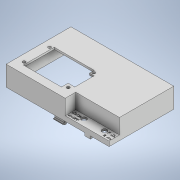
# Autodesk Inventor part: housing top
Saved by Autodesk Inventor 2020 (Build 240168000, 168)
## iProperties
Created: 2019-10-19
Part Number: housing top
Material: Generic
Document SubType Name: Modeling
Designer: strom
Density: 1 g/cm^3
Appearance: Default
Author: strom
Autodesk Inventor part; units mm, degrees
note: some values were not read from the file. Chosen so that the rebuilt part matches the saved one: direction of "Emboss1".
ref_plane "YZ Plane" through (0, 0, 0) normal (1, 0, 0) x (0, 1, 0)
ref_plane "XZ Plane" through (0, 0, 0) normal (0, 1, 0) x (-1, 0, 0)
sketch "Sketch1" plane through (0, 0, 0) normal (0, 1, 0) x (-1, 0, 0)
  line L0 (68.58, 43.18) -> (-68.58, 43.18)
  line L1 (-68.58, 43.18) -> (-68.58, -43.18)
  line L2 (-68.58, -43.18) -> (68.58, -43.18)
  line L3 (68.58, -43.18) -> (68.58, 43.18)
  line L4 (68.58, 43.18) -> (-68.58, -43.18) construction
  line L5 (-68.58, 43.18) -> (68.58, -43.18) construction
  point P0 (0, 0)
  dimension "d0" = 137.16
  dimension "d1" = 86.36
  constraints: 12 end point, 2 midpoint, 2 parallel, 1 horizontal, 1 perpendicular
  measures "d0" distance of L2.end L1.end
  measures "d1" distance of L1.end L0.end
extrude "Extrusion1" add sketch "Sketch1" along normal blind 25.4
sketch "Sketch2" plane through (0, 25.4, 0) normal (0, 1, 0) x (1, 0, 0)
  line L0 (-68.58, -43.18) -> (68.58, -43.18) projected
  line L1 (68.58, -43.18) -> (10.16, -43.18)
  line L2 (10.16, -43.18) -> (10.16, -29.21)
  line L3 (10.16, -29.21) -> (68.58, -29.21)
  line L4 (68.58, -29.21) -> (68.58, -43.18)
  point P0 (0, 0)
  dimension "d4" = 58.42
  dimension "d5" = 13.97
  constraints: 8 end point, 2 parallel, 1 horizontal, 1 perpendicular
  measures "d4" distance of L2.end L3.end
  measures "d5" distance of L1.end L2.end
extrude "Extrusion2" cut sketch "Sketch2" against normal blind 20.193
shell "Shell1" thickness 2.54 removed faces 1 at (-22.86, 0, -14.3933)
sketch "Sketch3" plane through (0, 0, 0) normal (0, -1, 0) x (1, 0, 0)
  line L0 (66.04, 40.64) -> (66.04, -40.64) projected
  line L1 (66.04, -40.64) -> (-66.04, -40.64) projected
  line L2 (-66.04, -40.64) -> (-66.04, 40.64) projected
  line L3 (-66.04, 40.64) -> (66.04, 40.64) projected
  line L4 (68.58, -43.18) -> (-68.58, -43.18) projected
  line L5 (68.58, 43.18) -> (68.58, -43.18) projected
  line L6 (-68.58, 43.18) -> (68.58, 43.18) projected
  line L7 (-68.58, -43.18) -> (-68.58, 43.18) projected
  line L8 (67.31, -41.91) -> (-67.31, -41.91)
  line L9 (-67.31, -41.91) -> (-67.31, 41.91)
  line L10 (-67.31, 41.91) -> (67.31, 41.91)
  line L11 (67.31, 41.91) -> (67.31, -41.91)
  line L12 (67.31, -41.91) -> (-67.31, 41.91) construction
  line L13 (-67.31, -41.91) -> (67.31, 41.91) construction
  point P0 (0, 0)
  dimension "d9" = 1.27
  dimension "d10" = 1.27
  constraints: 12 end point, 2 midpoint, 2 parallel, 1 horizontal, 1 perpendicular
  measures "d9" distance between parallel lines of L9 L2
  measures "d10" distance between parallel lines of L6 L10
extrude "Extrusion3" add sketch "Sketch3" along normal blind 1.27 contours L4 L7 L6 L5
sketch "Sketch4" plane through (0, -1.27, 0) normal (0, -1, 0) x (1, 0, 0)
  line L0 (68.58, 43.18) -> (-68.58, 43.18) projected
  line L1 (-66.04, 40.64) -> (66.04, 40.64) projected
  line L2 (36.449, 43.18) -> (43.688, 43.18)
  line L3 (43.688, 43.18) -> (43.688, 40.64)
  line L4 (43.688, 40.64) -> (36.449, 40.64)
  line L5 (36.449, 40.64) -> (36.449, 43.18)
  line L6 (68.58, -43.18) -> (68.58, 43.18) projected
  point P0 (0, 0)
  dimension "d13" = 24.892
  dimension "d14" = 7.239
  constraints: 8 end point, 2 parallel, 2 point on line, 1 horizontal, 1 perpendicular
  measures "d13" distance from line of L6 L3.end
  measures "d14" distance between parallel lines of L3 L5
extrude "Extrusion4" add sketch "Sketch4" along normal blind 3.81 and the other way blind 1.27
sketch "Sketch5" plane through (0, 0, 0) normal (1, 0, 0) x (0, 1, 0)
  line L0 (0, 40.64) -> (22.86, 40.64) projected
  line L1 (22.86, 40.64) -> (22.86, 37.846)
  line L2 (22.86, 40.64) -> (25.654, 40.64) construction
  line L3 (22.86, 37.846) -> (-8.89, 37.846)
  line L4 (-8.89, 37.846) -> (-8.89, 40.132)
  line L5 (-8.89, 40.132) -> (-7.2004, 42.545)
  line L6 (-7.2004, 42.545) -> (-6.35, 42.545)
  line L7 (-6.35, 42.545) -> (-6.35, 40.386)
  line L8 (-6.35, 40.386) -> (0, 40.386)
  line L9 (0, -40.64) -> (0, 40.64) projected
  line L10 (-1.27, 43.18) -> (25.4, 43.18) projected
  line L11 (-1.27, 43.18) -> (-1.27, -43.18) projected
  line L12 (0, 41.91) -> (0, -41.91) projected
  line L13 (22.86, -40.64) -> (22.86, 40.64) projected
  point P0 (0, 0)
  dimension "d21" = 2.54
  dimension "d22" = 0.254
  dimension "d23" = 35
  dimension "d25" = 5.08
  dimension "d26" = 2.54
  dimension "d31" = 0.508
  dimension "d32" = 1.905
  constraints: 16 end point, 3 perpendicular, 2 parallel, 2 point on line, 1 collinear, 1 horizontal, 1 vertical
  measures "d21" distance between parallel lines of L3 L8
  measures "d22" distance between parallel lines of L0 L8
  measures "d23" angle of L4 L5
  measures "d25" distance between parallel lines of L11 L7
  measures "d26" distance between parallel lines of L7 L4
  measures "d31" distance from line of L0 L4.end
  measures "d32" distance between parallel lines of L6 L0
extrude "Extrusion5" add sketch "Sketch5" along normal mid plane 12.7
ref_plane "Work Plane1" through (33.274, 5.207, 29.21) normal (1, 0, 0) x (0, 0, -1)
sketch "Sketch6" plane through (33.274, 5.207, 29.21) normal (1, 0, 0) x (0, 0, -1)
  line L0 (-13.97, -6.477) -> (-13.97, 20.193) projected
  line L1 (72.39, 20.193) -> (-13.97, 20.193) projected
  line L2 (72.39, -6.477) -> (72.39, 20.193) projected
  line L3 (-13.97, -6.477) -> (72.39, -6.477) projected
  line L4 (-12.7, -5.207) -> (71.12, -5.207) projected
  line L5 (71.12, -5.207) -> (71.12, -6.477) projected
  line L6 (69.85, -5.207) -> (69.85, 17.653) projected
  line L7 (67.056, 17.653) -> (67.056, -14.097)
  line L8 (67.056, -14.097) -> (69.342, -14.097)
  line L9 (69.342, -14.097) -> (71.755, -12.4074)
  line L10 (71.755, -12.4074) -> (71.755, -11.5692)
  line L11 (71.755, -11.5692) -> (69.596, -11.5692)
  line L12 (69.596, -11.5692) -> (69.596, -5.207)
  line L13 (69.85, 17.653) -> (-11.43, 17.653) projected
  point P0 (29.21, -5.207)
  dimension "d34" = 0.254
  dimension "d35" = 35
  dimension "d36" = 2.794
  dimension "d38" = 2.286
  dimension "d39" = 4.699
  dimension "d40" = 0.8382
  dimension "d41" = 31.75
  constraints: 12 end point, 3 perpendicular, 2 point on line, 1 parallel, 1 vertical
  measures "d34" distance between parallel lines of L6 L12
  measures "d35" angle of L8 L9
  measures "d36" distance between parallel lines of L7 L6
  measures "d38" distance of L7.end L8.end
  measures "d39" distance between parallel lines of L10 L7
  measures "d40" distance of L9.end L10.end
  measures "d41" distance of L7.start L7.end
extrude "Extrusion6" add sketch "Sketch6" along normal mid plane 12.7 contours L7 L4 L12 L3 | L3 L12 L11 L10 L9 L8 L7 | L7 L13 L6 L4
sketch "Sketch7" plane through (0, 5.207, 0) normal (0, 1, 0) x (1, 0, 0)
  line L0 (68.58, -29.21) -> (68.58, -43.18) projected
  line L1 (10.16, -29.21) -> (68.58, -29.21) projected
  line L2 (10.16, -43.18) -> (10.16, -29.21) projected
  line L3 (68.58, -43.18) -> (10.16, -43.18) projected
  circle A0 centre (26.416, -34.3535) radius 3.2385
  circle A1 centre (53.721, -34.3535) radius 3.2385
  line L4 (68.58, -43.18) -> (10.16, -43.18) projected
  line L5 (36.449, -43.18) -> (36.449, -40.64) projected
  line L6 (36.449, -40.64) -> (43.688, -40.64) projected
  line L7 (43.688, -40.64) -> (43.688, -43.18) projected
  line L8 (43.688, -43.18) -> (36.449, -43.18) projected
  point P0 (0, 0)
  dimension "d44" = 6.477
  dimension "d45" = 6.477
  dimension "d46" = 27.305
  dimension "d47" = 10.033
  dimension "d48" = 8.8265
  constraints: 2 centre point, 1 horizontal alignment
  measures "d44" diameter of A0
  measures "d45" diameter of A1
  measures "d46" distance of A1.centre A0.centre
  measures "d47" distance from line of A1.centre L7
  measures "d48" distance from line of L3 A1.centre
extrude "Extrusion7" cut sketch "Sketch7" against normal blind 12.7 contours A0 | A1
sketch "Sketch8" plane through (0, 25.4, 0) normal (0, 1, 0) x (1, 0, 0)
  line L0 (10.16, -43.18) -> (10.16, -29.21) projected
  line L1 (10.16, -29.21) -> (68.58, -29.21) projected
  line L2 (68.58, -29.21) -> (68.58, 43.18) projected
  line L3 (68.58, 43.18) -> (-68.58, 43.18) projected
  line L4 (-68.58, 43.18) -> (-68.58, -43.18) projected
  line L5 (-68.58, -43.18) -> (10.16, -43.18) projected
  line L6 (-66.04, -40.64) -> (-6.35, -40.64) projected
  line L7 (39.624, 37.846) -> (39.624, 40.64) projected
  line L8 (66.04, 40.64) -> (39.624, 40.64) projected
  line L9 (66.04, -26.67) -> (66.04, 40.64) projected
  line L10 (7.62, -26.67) -> (66.04, -26.67) projected
  line L11 (7.62, -40.64) -> (7.62, -26.67) projected
  line L12 (6.35, -40.64) -> (7.62, -40.64) projected
  line L13 (6.35, -40.64) -> (6.35, -37.846) projected
  line L14 (6.35, -37.846) -> (-6.35, -37.846) projected
  line L15 (-6.35, -37.846) -> (-6.35, -40.64) projected
  line L16 (-66.04, -40.64) -> (-6.35, -40.64) projected
  line L17 (-66.04, 40.64) -> (-66.04, -40.64) projected
  line L18 (26.924, 40.64) -> (-66.04, 40.64) projected
  line L19 (26.924, 40.64) -> (26.924, 37.846) projected
  line L20 (26.924, 37.846) -> (39.624, 37.846) projected
  line L21 (-64.77, 9.652) -> (4.826, 9.652)
  line L22 (4.826, 9.652) -> (4.826, -34.036)
  line L23 (4.826, -34.036) -> (-64.77, -34.036)
  line L24 (-64.77, -34.036) -> (-64.77, 9.652)
  line L25 (-56.134, 9.652) -> (-56.134, -34.036)
  line L26 (-2.794, 9.652) -> (-2.794, 2.032)
  line L27 (-2.794, 2.032) -> (4.826, 2.032)
  line L28 (-5.334, -34.036) -> (-5.334, -23.876)
  line L29 (-5.334, -23.876) -> (4.826, -23.876)
  line L30 (-5.334, -32.766) -> (-56.134, -32.766)
  line L31 (-56.134, 8.382) -> (-2.794, 8.382)
  line L32 (3.556, 2.032) -> (3.556, -23.876)
  point P0 (0, 0)
  dimension "d51" = 3.81
  dimension "d52" = 3.81
  dimension "d53" = 43.688
  dimension "d54" = 69.596
  dimension "d55" = 8.636
  dimension "d56" = 1.27
  dimension "d57" = 1.27
  dimension "d58" = 10.16
  dimension "d59" = 10.16
  dimension "d60" = 1.27
  dimension "d61" = 7.62
  dimension "d62" = 7.62
  constraints: 24 end point, 12 point on line, 7 perpendicular, 2 parallel, 2 vertical, 1 horizontal
  measures "d51" distance between parallel lines of L4 L24
  measures "d52" distance between parallel lines of L23 L14
  measures "d53" distance between parallel lines of L21 L23
  measures "d54" distance between parallel lines of L22 L24
  measures "d55" distance between parallel lines of L24 L25
  measures "d56" distance between parallel lines of L21 L31
  measures "d57" distance between parallel lines of L23 L30
  measures "d58" distance between parallel lines of L23 L29
  measures "d59" distance between parallel lines of L28 L22
  measures "d60" distance between parallel lines of L32 L22
  measures "d61" distance between parallel lines of L27 L21
  measures "d62" distance between parallel lines of L22 L26
extrude "Extrusion8" cut sketch "Sketch8" against normal blind 12.7 contours L31 L26 L27 L32 L29 L28 L30 L25
sketch "Sketch9" plane through (0, 25.4, 0) normal (0, 1, 0) x (1, 0, 0)
  circle A0 centre (-0.254, 5.207) radius 1.905
  circle A1 centre (-0.254, -28.829) radius 1.905
  circle A2 centre (-59.182, -28.829) radius 1.905
  circle A3 centre (-59.182, 5.207) radius 1.905
  line L0 (-2.794, 2.032) -> (3.556, 2.032) projected
  line L1 (-2.794, 8.382) -> (-2.794, 2.032) projected
  point P0 (0, 0)
  dimension "d65" = 3.81
  dimension "d66" = 3.81
  dimension "d67" = 3.81
  dimension "d68" = 3.81
  dimension "d69" = 58.928
  dimension "d70" = 34.036
  dimension "d71" = 3.175
  dimension "d72" = 2.54
  constraints: 4 centre point, 2 horizontal alignment, 2 vertical alignment
  measures "d65" diameter of A3
  measures "d66" diameter of A2
  measures "d67" diameter of A0
  measures "d68" diameter of A1
  measures "d69" distance of A0.centre A3.centre
  measures "d70" distance of A2.centre A3.centre
  measures "d71" distance from line of A0.centre L0
  measures "d72" distance from line of A0.centre L1
extrude "Extrusion9" cut sketch "Sketch9" against normal blind 12.7
sketch "Sketch10" plane through (0, 5.207, 0) normal (0, 1, 0) x (1, 0, 0)
  line L0 (11.43, -34.29) -> (13.0175, -34.29)
  line L1 (13.0175, -34.29) -> (13.0175, -32.385)
  line L2 (13.0175, -32.385) -> (14.9225, -32.385)
  line L3 (14.9225, -32.385) -> (14.9225, -34.29)
  line L4 (14.9225, -34.29) -> (16.51, -34.29)
  line L5 (16.51, -34.29) -> (16.51, -35.56)
  line L6 (16.51, -35.56) -> (11.43, -35.56)
  line L7 (11.43, -35.56) -> (11.43, -34.29)
  line L8 (11.43, -40.8622) -> (16.51, -40.8622)
  line L9 (16.51, -40.8622) -> (16.51, -39.5922)
  line L10 (16.51, -39.5922) -> (14.9225, -39.5922)
  line L11 (14.9225, -39.5922) -> (14.9225, -39.116)
  line L12 (14.9225, -39.116) -> (13.0175, -39.116)
  line L13 (13.0175, -39.116) -> (13.0175, -39.5922)
  line L14 (13.0175, -39.5922) -> (11.43, -39.5922)
  line L15 (11.43, -40.8622) -> (11.43, -39.5922)
  line L16 (10.16, -43.18) -> (10.16, -29.21) projected
  line L17 (10.16, -29.21) -> (68.58, -29.21) projected
  line L18 (14.661, -39.3775) -> (14.661, -39.8537)
  line L19 (14.661, -39.8537) -> (16.2485, -39.8537)
  line L20 (16.2485, -39.8537) -> (16.2485, -40.6008)
  line L21 (16.2485, -40.6008) -> (11.6915, -40.6008)
  line L22 (11.6915, -40.6008) -> (11.6915, -39.8537)
  line L23 (11.6915, -39.8537) -> (13.279, -39.8537)
  line L24 (13.279, -39.8537) -> (13.279, -39.3775)
  line L25 (13.279, -39.3775) -> (14.661, -39.3775)
  line L26 (16.2537, -34.5463) -> (14.6662, -34.5463)
  line L27 (14.6662, -34.5463) -> (14.6662, -32.6413)
  line L28 (14.6662, -32.6413) -> (13.2738, -32.6413)
  line L29 (13.2738, -32.6413) -> (13.2738, -34.5463)
  line L30 (13.2738, -34.5463) -> (11.6863, -34.5463)
  line L31 (11.6863, -34.5463) -> (11.6863, -35.3037)
  line L32 (11.6863, -35.3037) -> (16.2537, -35.3037)
  line L33 (16.2537, -35.3037) -> (16.2537, -34.5463)
  line L34 (17.0101, -32.6962) -> (22.7751, -32.6962) construction
  line L35 (22.7751, -32.6962) -> (22.7751, -35.8726) construction
  line L36 (22.7751, -35.8726) -> (17.0101, -35.8726) construction
  line L37 (17.0101, -35.8726) -> (17.0101, -32.6962) construction
  line L38 (17.0101, -38.1814) -> (22.4449, -38.1814) construction
  line L39 (22.4449, -38.1814) -> (22.4449, -41.4779) construction
  line L40 (22.4449, -41.4779) -> (17.0101, -41.4779) construction
  line L41 (17.0101, -41.4779) -> (17.0101, -38.1814) construction
  line L42 (62.753, -34.29) -> (64.3405, -34.29)
  line L43 (64.3405, -34.29) -> (64.3405, -32.385)
  line L44 (64.3405, -32.385) -> (66.2455, -32.385)
  line L45 (66.2455, -32.385) -> (66.2455, -34.29)
  line L46 (66.2455, -34.29) -> (67.833, -34.29)
  line L47 (67.833, -34.29) -> (67.833, -35.56)
  line L48 (67.833, -35.56) -> (62.753, -35.56)
  line L49 (62.753, -35.56) -> (62.753, -34.29)
  line L50 (12.925, -32.9588) -> (11.3375, -32.9588)
  line L51 (66.2455, -39.116) -> (66.2455, -39.5922)
  line L52 (64.3405, -39.116) -> (66.2455, -39.116)
  line L53 (62.753, -40.8622) -> (62.753, -39.5922)
  line L54 (62.753, -39.5922) -> (64.3405, -39.5922)
  line L55 (67.833, -40.8622) -> (62.753, -40.8622)
  line L56 (66.2455, -39.5922) -> (67.833, -39.5922)
  line L57 (64.3405, -39.5922) -> (64.3405, -39.116)
  line L58 (67.833, -39.5922) -> (67.833, -40.8622)
  line L59 (67.579, -34.544) -> (65.9915, -34.544)
  line L60 (65.9915, -34.544) -> (65.9915, -32.639)
  line L61 (65.9915, -32.639) -> (64.5945, -32.639)
  line L62 (64.5945, -32.639) -> (64.5945, -34.544)
  line L63 (64.5945, -34.544) -> (63.007, -34.544)
  line L64 (63.007, -34.544) -> (63.007, -35.306)
  line L65 (63.007, -35.306) -> (67.579, -35.306)
  line L66 (67.579, -35.306) -> (67.579, -34.544)
  line L67 (67.579, -39.8462) -> (65.9915, -39.8462)
  line L68 (65.9915, -39.8462) -> (65.9915, -39.37)
  line L69 (65.9915, -39.37) -> (64.5945, -39.37)
  line L70 (64.5945, -39.37) -> (64.5945, -39.8462)
  line L71 (64.5945, -39.8462) -> (63.007, -39.8462)
  line L72 (63.007, -39.8462) -> (63.007, -40.6082)
  line L73 (63.007, -40.6082) -> (67.579, -40.6082)
  line L74 (67.579, -40.6082) -> (67.579, -39.8462)
  line L75 (58.0602, -32.1559) -> (60.2461, -32.1559) construction
  line L76 (60.2461, -32.1559) -> (60.2461, -35.2039) construction
  line L77 (60.2461, -35.2039) -> (58.0602, -35.2039) construction
  line L78 (58.0602, -35.2039) -> (58.0602, -32.1559) construction
  line L79 (58.0602, -38.2294) -> (60.6611, -38.2294) construction
  line L80 (60.6611, -38.2294) -> (60.6611, -41.2774) construction
  line L81 (60.6611, -41.2774) -> (58.0602, -41.2774) construction
  line L82 (58.0602, -41.2774) -> (58.0602, -38.2294) construction
  spline S0 degree 2 poles (19.4752, -33.1087) (19.6481, -33.3112) (19.8407, -33.904) (19.8407, -34.2844) knots 0 0 0 1 2 2 2
  spline S1 degree 2 poles (19.8407, -34.2844) (19.8407, -34.6549) (19.653, -35.2551) (19.4752, -35.4576) knots 0 0 0 1 2 2 2
  spline S2 degree 2 poles (19.4752, -35.4576) (19.2875, -35.6701) (18.791, -35.8726) (18.4921, -35.8726) knots 0 0 0 1 2 2 2
  spline S3 degree 2 poles (18.4921, -35.8726) (18.1834, -35.8726) (17.6894, -35.6627) (17.5091, -35.4576) knots 0 0 0 1 2 2 2
  spline S4 degree 2 poles (17.5091, -35.4576) (17.3337, -35.2551) (17.146, -34.6598) (17.146, -34.2844) knots 0 0 0 1 2 2 2
  spline S5 degree 2 poles (17.146, -34.2844) (17.146, -33.9015) (17.3361, -33.3186) (17.5115, -33.1087) knots 0 0 0 1 2 2 2
  spline S6 degree 2 poles (17.5115, -33.1087) (17.6894, -32.9061) (18.1858, -32.6962) (18.4921, -32.6962) knots 0 0 0 1 2 2 2
  spline S7 degree 2 poles (18.4921, -32.6962) (18.8033, -32.6962) (19.3023, -32.9135) (19.4752, -33.1087) knots 0 0 0 1 2 2 2
  spline S8 degree 2 poles (19.4184, -34.2844) (19.4184, -33.983) (19.2875, -33.5162) (19.1689, -33.3631) knots 0 0 0 1 2 2 2
  spline S9 degree 2 poles (19.1689, -33.3631) (19.0479, -33.205) (18.707, -33.0469) (18.4946, -33.0469) knots 0 0 0 1 2 2 2
  spline S10 degree 2 poles (18.4946, -33.0469) (18.2748, -33.0469) (17.9438, -33.2001) (17.8178, -33.3631) knots 0 0 0 1 2 2 2
  spline S11 degree 2 poles (17.8178, -33.3631) (17.6968, -33.5187) (17.5683, -33.988) (17.5683, -34.2844) knots 0 0 0 1 2 2 2
  spline S12 degree 2 poles (17.5683, -34.2844) (17.5683, -34.8846) (18.0722, -35.5219) (18.4946, -35.5219) knots 0 0 0 1 2 2 2
  spline S13 degree 2 poles (18.4946, -35.5219) (18.917, -35.5219) (19.4184, -34.8846) (19.4184, -34.2844) knots 0 0 0 1 2 2 2
  line L83 (22.4664, -35.8084) -> (22.0119, -35.8084)
  line L84 (22.0119, -35.8084) -> (20.6633, -33.1803)
  line L85 (20.6633, -33.1803) -> (20.6633, -35.8084)
  line L86 (20.6633, -35.8084) -> (20.2853, -35.8084)
  line L87 (20.2853, -35.8084) -> (20.2853, -32.7604)
  line L88 (20.2853, -32.7604) -> (20.8609, -32.7604)
  line L89 (20.8609, -32.7604) -> (22.0885, -35.1736)
  line L90 (22.0885, -35.1736) -> (22.0885, -32.7604)
  line L91 (22.0885, -32.7604) -> (22.4664, -32.7604)
  line L92 (22.4664, -32.7604) -> (22.4664, -35.8084)
  spline S14 degree 2 poles (19.4752, -38.5939) (19.6481, -38.7964) (19.8407, -39.3892) (19.8407, -39.7696) knots 0 0 0 1 2 2 2
  spline S15 degree 2 poles (19.8407, -39.7696) (19.8407, -40.1401) (19.653, -40.7403) (19.4752, -40.9429) knots 0 0 0 1 2 2 2
  spline S16 degree 2 poles (19.4752, -40.9429) (19.2875, -41.1553) (18.791, -41.3578) (18.4921, -41.3578) knots 0 0 0 1 2 2 2
  spline S17 degree 2 poles (18.4921, -41.3578) (18.1834, -41.3578) (17.6894, -41.1479) (17.5091, -40.9429) knots 0 0 0 1 2 2 2
  spline S18 degree 2 poles (17.5091, -40.9429) (17.3337, -40.7403) (17.146, -40.1451) (17.146, -39.7696) knots 0 0 0 1 2 2 2
  spline S19 degree 2 poles (17.146, -39.7696) (17.146, -39.3868) (17.3361, -38.8038) (17.5115, -38.5939) knots 0 0 0 1 2 2 2
  spline S20 degree 2 poles (17.5115, -38.5939) (17.6894, -38.3913) (18.1858, -38.1814) (18.4921, -38.1814) knots 0 0 0 1 2 2 2
  spline S21 degree 2 poles (18.4921, -38.1814) (18.8033, -38.1814) (19.3023, -38.3988) (19.4752, -38.5939) knots 0 0 0 1 2 2 2
  spline S22 degree 2 poles (19.4184, -39.7696) (19.4184, -39.4683) (19.2875, -39.0014) (19.1689, -38.8483) knots 0 0 0 1 2 2 2
  spline S23 degree 2 poles (19.1689, -38.8483) (19.0479, -38.6902) (18.707, -38.5321) (18.4946, -38.5321) knots 0 0 0 1 2 2 2
  spline S24 degree 2 poles (18.4946, -38.5321) (18.2748, -38.5321) (17.9438, -38.6853) (17.8178, -38.8483) knots 0 0 0 1 2 2 2
  spline S25 degree 2 poles (17.8178, -38.8483) (17.6968, -39.0039) (17.5683, -39.4732) (17.5683, -39.7696) knots 0 0 0 1 2 2 2
  spline S26 degree 2 poles (17.5683, -39.7696) (17.5683, -40.3698) (18.0722, -41.0071) (18.4946, -41.0071) knots 0 0 0 1 2 2 2
  spline S27 degree 2 poles (18.4946, -41.0071) (18.917, -41.0071) (19.4184, -40.3698) (19.4184, -39.7696) knots 0 0 0 1 2 2 2
  line L93 (22.1082, -38.6062) -> (20.6904, -38.6062)
  line L94 (20.6904, -38.6062) -> (20.6904, -39.4658)
  line L95 (20.6904, -39.4658) -> (22.0489, -39.4658)
  line L96 (22.0489, -39.4658) -> (22.0489, -39.8264)
  line L97 (22.0489, -39.8264) -> (20.6904, -39.8264)
  line L98 (20.6904, -39.8264) -> (20.6904, -41.2936)
  line L99 (20.6904, -41.2936) -> (20.2853, -41.2936)
  line L100 (20.2853, -41.2936) -> (20.2853, -38.2456)
  line L101 (20.2853, -38.2456) -> (22.1082, -38.2456)
  line L102 (22.1082, -38.2456) -> (22.1082, -38.6062)
  line L103 (24.2942, -38.6062) -> (22.8764, -38.6062)
  line L104 (22.8764, -38.6062) -> (22.8764, -39.4658)
  line L105 (22.8764, -39.4658) -> (24.2349, -39.4658)
  line L106 (24.2349, -39.4658) -> (24.2349, -39.8264)
  line L107 (24.2349, -39.8264) -> (22.8764, -39.8264)
  line L108 (22.8764, -39.8264) -> (22.8764, -41.2936)
  line L109 (22.8764, -41.2936) -> (22.4713, -41.2936)
  line L110 (22.4713, -41.2936) -> (22.4713, -38.2456)
  line L111 (22.4713, -38.2456) -> (24.2942, -38.2456)
  line L112 (24.2942, -38.2456) -> (24.2942, -38.6062)
  line L113 (60.1918, -32.5165) -> (58.774, -32.5165)
  line L114 (58.774, -32.5165) -> (58.774, -33.376)
  line L115 (58.774, -33.376) -> (60.1325, -33.376)
  line L116 (60.1325, -33.376) -> (60.1325, -33.7367)
  line L117 (60.1325, -33.7367) -> (58.774, -33.7367)
  line L118 (58.774, -33.7367) -> (58.774, -35.2039)
  line L119 (58.774, -35.2039) -> (58.3689, -35.2039)
  line L120 (58.3689, -35.2039) -> (58.3689, -32.1559)
  line L121 (58.3689, -32.1559) -> (60.1918, -32.1559)
  line L122 (60.1918, -32.1559) -> (60.1918, -32.5165)
  line L123 (60.7278, -41.2774) -> (60.2017, -41.2774)
  line L124 (60.2017, -41.2774) -> (59.2384, -40.0647)
  line L125 (59.2384, -40.0647) -> (58.774, -40.0647)
  line L126 (58.774, -40.0647) -> (58.774, -41.2774)
  line L127 (58.774, -41.2774) -> (58.3689, -41.2774)
  line L128 (58.3689, -41.2774) -> (58.3689, -38.2294)
  line L129 (58.3689, -38.2294) -> (59.1544, -38.2294)
  spline S28 degree 2 poles (59.1544, -38.2294) (59.4162, -38.2294) (59.7694, -38.2863) (59.93, -38.39) knots 0 0 0 1 2 2 2
  spline S29 degree 2 poles (59.93, -38.39) (60.0905, -38.4937) (60.2758, -38.8173) (60.2758, -39.0569) knots 0 0 0 1 2 2 2
  spline S30 degree 2 poles (60.2758, -39.0569) (60.2758, -39.3904) (59.9349, -39.8424) (59.6434, -39.951) knots 0 0 0 1 2 2 2
  line L130 (59.6434, -39.951) -> (60.7278, -41.2774)
  spline S31 degree 2 poles (59.8534, -39.089) (59.8534, -38.9556) (59.7595, -38.7506) (59.6607, -38.6839) knots 0 0 0 1 2 2 2
  spline S32 degree 2 poles (59.6607, -38.6839) (59.5743, -38.6271) (59.3446, -38.5802) (59.1766, -38.5802) knots 0 0 0 1 2 2 2
  line L131 (59.1766, -38.5802) -> (58.774, -38.5802)
  line L132 (58.774, -38.5802) -> (58.774, -39.7263)
  line L133 (58.774, -39.7263) -> (59.1297, -39.7263)
  spline S33 degree 2 poles (59.1297, -39.7263) (59.305, -39.7263) (59.5842, -39.6645) (59.6805, -39.5682) knots 0 0 0 1 2 2 2
  spline S34 degree 2 poles (59.6805, -39.5682) (59.7694, -39.4842) (59.8534, -39.2471) (59.8534, -39.089) knots 0 0 0 1 2 2 2
  point P0 (0, 0)
  point P1 (13.0175, -39.3541)
  point P2 (62.753, -39.2747)
  point P3 (67.833, -39.2747)
  point P4 (67.833, -38.0047)
  point P5 (64.3405, -37.5285)
  point P6 (62.753, -38.0047)
  point P7 (62.753, -37.6872)
  point P8 (62.753, -36.4172)
  point P9 (64.3405, -35.941)
  point P10 (67.833, -37.6872)
  point P11 (67.833, -36.4172)
  dimension "d75" = 5.08
  dimension "d76" = 1.905
  dimension "d77" = 1.905
  dimension "d78" = 1.27
  dimension "d79" = 1.27
  dimension "d80" = 1.905
  dimension "d81" = 0.4763
  dimension "d82" = 3.556
  dimension "d84" = 3.175
  dimension "d85" = 5.08
  dimension "d86" = 1.905
  dimension "d87" = 1.27
  dimension "d88" = 1.905
  dimension "d89" = 5.08
  dimension "d90" = 1.905
  dimension "d91" = 1.27
  dimension "d92" = 0.4763
  dimension "d93" = 3.175
  dimension "d94" = 3.556
  dimension "d95" = 0.254
  dimension "d96" = 0.254
  constraints: 130 end point, 45 perpendicular, 23 point on line, 6 collinear, 3 horizontal, 3 vertical, 1 midpoint, 36 other
  measures "d75" distance between parallel lines of L5 L7
  measures "d76" distance between parallel lines of L3 L1
  measures "d77" distance between parallel lines of L11 L13
  measures "d78" distance between parallel lines of L6 L0
  measures "d79" distance between parallel lines of L8 L14
  measures "d80" distance between parallel lines of L0 L2
  measures "d81" distance between parallel lines of L14 L12
  measures "d82" distance between parallel lines of L12 L6
  measures "d84" distance between parallel lines of L2 L17
  measures "d85" distance between parallel lines of L47 L49
  measures "d86" distance between parallel lines of L45 L43
  measures "d87" distance between parallel lines of L48 L42
  measures "d88" distance between parallel lines of L42 L44
  measures "d89" distance between parallel lines of L58 L53
  measures "d90" distance between parallel lines of L51 L57
  measures "d91" distance between parallel lines of L55 L54
  measures "d92" distance between parallel lines of L54 L52
  measures "d93" distance between parallel lines of L44 L17
  measures "d94" distance between parallel lines of L52 L48
  measures "d95" distance between parallel lines of L46 L59
  measures "d96" distance between parallel lines of L56 L67
emboss "Emboss1" sketch "Sketch10" operation cut depth 1.905 direction (0, -1, 0)
equation "\"d45\" = d44"
equation "\"d66\" = d65"
equation "\"d67\" = d65"
equation "\"d68\" = d65"
equation "\"d77\" = d76"
equation "\"d79\" = d78"
equation "\"d81\" = 0.25 * d80"
equation "\"d92\" = 0.25 * d88"
body "Solid1"
